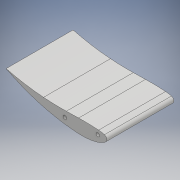
# Autodesk Inventor part: main flap
Saved by Autodesk Inventor 2018.3 (Build 223284000, 284)
## iProperties
Created: 2018-06-13
Part Number: main flap
Material: 一般
Document SubType Name: Modeling
Designer: ku_sk
Density: 1 g/cm^3
Appearance: 既定
Author: ku_sk
Autodesk Inventor part; units mm, degrees
ref_plane "YZ Plane" through (0, 0, 0) normal (1, 0, 0) x (0, 1, 0)
ref_plane "XZ Plane" through (0, 0, 0) normal (0, 1, 0) x (-1, 0, 0)
ref_plane "XY Plane" through (0, 0, 0) normal (0, 0, 1) x (1, 0, 0)
sketch "スケッチ1" plane through (0, 0, 0) normal (0, 1, 0) x (-1, 0, 0)
  arc A0 (101.7324, -28.9004) -> (328.1926, 37.3714) centre (48.6916, 572.4065) ccw projected
  arc A1 (202.438, 16.5387) -> (328.1926, 37.3714) centre (148.7903, 730.3461) ccw projected
  arc A2 (125.7464, 14.4013) -> (202.438, 16.5387) centre (141.4444, 828.0876) ccw projected
  arc A3 (84.4867, 15.2639) -> (125.7464, 14.4013) centre (372.4747, 12803.2702) ccw projected
  arc A4 (84.4867, 15.2639) -> (17.3799, 13.5681) centre (68.6653, -687.2803) ccw projected
  arc A5 (17.3799, 13.5681) -> (-2.611, 10.3374) centre (25.867, -102.4131) ccw projected
  arc A6 (-2.611, 10.3374) -> (-8.1443, -6.881) centre (0, 0) ccw projected
  arc A7 (-8.1443, -6.881) -> (0.1105, -13.8465) centre (16.4695, 13.9147) ccw projected
  arc A8 (0.1105, -13.8465) -> (28.2747, -25.3165) centre (53.2618, 76.3513) ccw projected
  arc A9 (28.2747, -25.3165) -> (76.0298, -30.4027) centre (70.8911, 148.0818) ccw projected
  arc A10 (76.0298, -30.4027) -> (101.7324, -28.9004) centre (63.5115, 404.3974) ccw projected
  circle A11 centre (20.1088, -0.8575) radius 6 projected
  circle A12 centre (130.7072, -5.574) radius 6 projected
  point P0 (0, 0)
extrude "押し出し1" add sketch "スケッチ1" along normal mid plane 225
